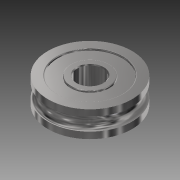
# Autodesk Inventor part: bearing_604uu
Saved by Autodesk Inventor 2013 (Build 170138000, 138)
## iProperties
Created: 2015-02-20
Part Number: bearing_604uu
Material: 一般
Document SubType Name: Modeling
Designer: Noa Izumi
Density: 1 g/cm^3
Author: Noa Izumi
Autodesk Inventor part; units mm, degrees
ref_plane "YZ Plane" through (0, 0, 0) normal (1, 0, 0) x (0, 1, 0)
ref_plane "XZ Plane" through (0, 0, 0) normal (0, 1, 0) x (-1, 0, 0)
ref_plane "XY Plane" through (0, 0, 0) normal (0, 0, 1) x (1, 0, 0)
sketch "草圖1" plane through (0, 0, 0) normal (0, 1, 0) x (-1, 0, 0)
  line L0 (0, 0) -> (6.5, 0)
  line L1 (6.5, 4) -> (0, 4)
  line L2 (0, 4) -> (0, 0)
  arc A0 (6.5, 3) -> (6.5, 1) centre (6.5, 2) ccw
  line L3 (6.5, 0) -> (6.5, 1)
  line L4 (6.5, 3) -> (6.5, 4)
  line L5 (3, 4) -> (5, 4)
  line L6 (5, 4) -> (5, 3.75)
  line L7 (5, 3.75) -> (3, 3.75)
  line L8 (3, 3.75) -> (3, 4)
  line L9 (3, 0) -> (5, 0)
  line L10 (5, 0) -> (5, 0.2496)
  line L11 (5, 0.2496) -> (3, 0.2496)
  line L12 (3, 0.2496) -> (3, 0)
  dimension "d2" = 6.5
  dimension "d4" = 4
  dimension "d5" = 2
  dimension "d7" = 3
  dimension "d8" = 1.5
  dimension "d9" = 0.25
  dimension "d10" = 0.2495
  constraints: 26 end point, 7 parallel, 4 perpendicular, 3 horizontal, 2 point on circle, 2 point on line, 1 centre point
  measures "d2" distance of L1.start L1.end
  measures "d4" distance of L1.end L0.start
  measures "d5" diameter of A0
  measures "d7" distance between parallel lines of L2 L8
  measures "d8" distance between parallel lines of L4 L6
  measures "d9" distance between parallel lines of L7 L1
  measures "d10" distance of L9.end L10.end
revolve "迴轉2" add sketch "草圖1" angle 360 about axis through (0, 0, 4) along (0, 0, -1) contours L2 L1 L8 L7 L6 L4 A0 L3 L0 L10 L11 L12
sketch "草圖2" plane through (0, 0, 4) normal (0, 0, 1) x (1, 0, 0)
  circle A0 centre (0, 0) radius 3 projected
  constraints: 1 coincident
hole "孔1" at (0, 0, 4) direction (0, 0, -1) diameter 4 end through all
chamfer "倒角1" distance 0.125 angle 45 2 edges at (0, 2, 4) (0, 2, 0)
fillet "圓角2" radius 0.125 4 edges at (3, 0, 4) (5, 0, 4) (5, 0, 0) (3, 0, 0)
